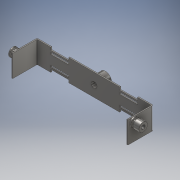
# Autodesk Inventor part: Maintient courvercle
Saved by Autodesk Inventor 2017 (Build 210142000, 142)
## iProperties
Company: FABLAB Frenchmakers
Part Number: Maintient courvercle
Material: Acier inoxydable
Document SubType Name: Modeling
Designer: FABLAB Frenchmakers
Density: 8 g/cm^3
Appearance: Semi-poli
Mass: 121.443 g
Surface Area: 157.681 cm^2
Volume: 15.1804 cm^3
Project: 1400-PopCorn Machine
Stock Number: 1400-01-03
Author: Adrien MARY
Autodesk Inventor part; units mm, degrees
sketch "Esquisse1" plane through (0, 0, 0) normal (0, 0, 1) x (1, 0, 0)
  line L0 (-80, 0) -> (-80, 35)
  line L1 (-80, 35) -> (80, 35)
  line L2 (80, 35) -> (80, 0)
  line L3 (80, 0) -> (78.5, 0)
  line L4 (78.5, 0) -> (78.5, 33.5)
  line L5 (78.5, 33.5) -> (-78.5, 33.5)
  line L6 (-78.5, 33.5) -> (-78.5, 0)
  line L7 (-78.5, 0) -> (-80, 0)
  point P0 (0, 0)
  point P1 (-79.25, 0)
  point P2 (0, 35)
  point P3 (0, 33.5)
  dimension "d0" = 1.5
  dimension "d1" = 1.5
  dimension "d2" = 160
  dimension "d3" = 35
  constraints: 16 end point, 4 vertical, 3 horizontal, 3 midpoint, 2 vertical alignment, 1 collinear, 1 horizontal alignment, 1 perpendicular
  measures "d0" distance between parallel lines of L2 L4
  measures "d1" distance between parallel lines of L1 L5
  measures "d2" distance between parallel lines of L2 L0
  measures "d3" distance between parallel lines of L3 L1
extrude "Extrusion1" add sketch "Esquisse1" along normal mid plane 30
fillet "Congé1" radius 2 2 edges at (80, 35, 0) (-80, 35, 0)
fillet "Congé1" radius 1 2 edges at (-78.5, 33.5, 0) (78.5, 33.5, 0)
sketch "Esquisse2" plane through (-78, 35, 15) normal (0, 1, 0) x (1, 0, 0)
  line L0 (64.3632, 4.6) -> (91.6368, 4.6)
  line L1 (91.6368, 25.4) -> (64.3632, 25.4)
  arc A0 (64.3632, 25.4) -> (64.3632, 4.6) centre (78, 15) ccw
  arc A1 (91.6368, 4.6) -> (91.6368, 25.4) centre (78, 15) ccw
  point P0 (102.0926, 15)
  dimension "d9" = 20.8
  dimension "d10" = 17.15
  dimension "d11" = 17.15
  dimension "d12" = 10.4
  constraints: 4 end point, 4 point on circle, 2 centre point, 1 coincident, 1 horizontal, 1 horizontal alignment, 1 parallel
  measures "d9" distance between parallel lines of L1 L0
  measures "d10" radius of A1
  measures "d11" radius of A0
  measures "d12" distance from line of point (78, 15) L1
extrude "Extrusion2" add sketch "Esquisse2" along normal blind 4
sketch "Esquisse3" plane through (-78, 39, 15) normal (0, 1, 0) x (1, 0, 0)
  circle A0 centre (78, 15) radius 8.75
  dimension "d15" = 17.5
  constraints: 1 centre point, 1 coincident
  measures "d15" diameter of A0
extrude "Extrusion3" add sketch "Esquisse3" along normal blind 10 draft -1.43
sketch "Esquisse6" plane through (-80, 0, -15) normal (-1, 0, 0) x (0, 0, 1)
  circle A0 centre (24, 8) radius 6
  line L0 (30, 33) -> (30, 0) projected
  point P0 (15, 0)
  dimension "d20" = 12
  dimension "d21" = 8
  constraints: 1 centre point, 1 tangent
  measures "d20" diameter of A0
  measures "d21" vertical distance of point (15, 0) A0.centre
extrude "Extrusion4" add sketch "Esquisse6" along normal blind 6.65
ref_plane "Plan de construction4" through (-84.65, 8, 9) normal (-1, 0, 0) x (0, 0, 1)
sketch "Esquisse7" plane through (-84.65, 8, 9) normal (-1, 0, 0) x (0, 0, 1)
  circle A0 centre (0, 0) radius 6 construction
  circle A1 centre (0, 0) radius 3.75
  circle A2 centre (0, 0) radius 7
  point P0 (-9, -8)
  point P1 (6, 0)
  dimension "d25" = 7.5
  dimension "d26" = 1
  constraints: 2 centre point, 2 coincident, 1 horizontal alignment
  measures "d25" diameter of A1
extrude "Extrusion5" cut sketch "Esquisse7" against normal blind 2.6
mirror "Symétrie2" about plane through (0, 0, 0) normal (1, 0, 0) of "Extrusion4", "Extrusion5"
sketch "Esquisse8" plane through (-78, 35, 15) normal (0, 1, 0) x (1, 0, 0)
  line L0 (18.2, 21.5) -> (43, 21.5)
  line L1 (43, 21.5) -> (43, 30)
  line L2 (43, 30) -> (18.2, 30)
  line L3 (18.2, 30) -> (18.2, 21.5)
  line L4 (113, 21.5) -> (137.8, 21.5)
  line L5 (137.8, 21.5) -> (137.8, 30)
  line L6 (137.8, 30) -> (113, 30)
  line L7 (113, 30) -> (113, 21.5)
  line L8 (113, 0) -> (137.8, 0)
  line L9 (137.8, 0) -> (137.8, 8.5)
  line L10 (137.8, 8.5) -> (113, 8.5)
  line L11 (113, 8.5) -> (113, 0)
  line L12 (18.2, 0) -> (43, 0)
  line L13 (43, 0) -> (43, 8.5)
  line L14 (43, 8.5) -> (18.2, 8.5)
  line L15 (18.2, 8.5) -> (18.2, 0)
  line L16 (0, 30) -> (156, 30) projected
  line L17 (156, 0) -> (0, 0) projected
  point P0 (78, 15)
  dimension "d32" = 24.8
  dimension "d33" = 24.8
  dimension "d34" = 70
  dimension "d35" = 35
  dimension "d36" = 8.5
  dimension "d37" = 8.5
  constraints: 32 end point, 8 collinear, 8 parallel, 4 horizontal, 4 perpendicular, 2 point on line
  measures "d32" distance of L13.end L14.end
  measures "d33" distance of L9.end L10.end
  measures "d34" distance between parallel lines of L7 L1
  measures "d35" distance from line of L1 point (78, 15)
  measures "d36" distance between parallel lines of L16 L0
  measures "d37" distance between parallel lines of L17 L14
extrude "Extrusion6" cut sketch "Esquisse8" against normal through all
sketch "Esquisse9" plane through (78, 35, 15) normal (0, 1, 0) x (1, 0, 0)
  line L0 (-137.8, 23.9) -> (-113, 23.9)
  line L1 (-113, 23.9) -> (-113, 26.4)
  line L2 (-113, 26.4) -> (-137.8, 26.4)
  line L3 (-137.8, 26.4) -> (-137.8, 23.9)
  line L4 (-137.8, 3.6) -> (-113, 3.6)
  line L5 (-113, 3.6) -> (-113, 6.1)
  line L6 (-113, 6.1) -> (-137.8, 6.1)
  line L7 (-137.8, 6.1) -> (-137.8, 3.6)
  line L8 (-43, 23.9) -> (-18.2, 23.9)
  line L9 (-18.2, 23.9) -> (-18.2, 26.4)
  line L10 (-18.2, 26.4) -> (-43, 26.4)
  line L11 (-43, 26.4) -> (-43, 23.9)
  line L12 (-43, 3.6) -> (-18.2, 3.6)
  line L13 (-18.2, 3.6) -> (-18.2, 6.1)
  line L14 (-18.2, 6.1) -> (-43, 6.1)
  line L15 (-43, 6.1) -> (-43, 3.6)
  line L16 (-137.8, 21.5) -> (-137.8, 30) projected
  line L17 (-113, 30) -> (-113, 21.5) projected
  line L18 (-43, 21.5) -> (-43, 30) projected
  line L19 (-18.2, 30) -> (-18.2, 21.5) projected
  line L20 (-113, 21.5) -> (-137.8, 21.5) projected
  line L21 (-137.8, 8.5) -> (-113, 8.5) projected
  point P0 (-78, 15)
  dimension "d40" = 2.5
  dimension "d41" = 2.5
  dimension "d42" = 2.4
  dimension "d43" = 2.4
  constraints: 32 end point, 11 collinear, 8 parallel, 4 horizontal, 4 perpendicular, 1 point on line
  measures "d40" distance between parallel lines of L2 L0
  measures "d41" distance between parallel lines of L6 L4
  measures "d42" distance between parallel lines of L20 L0
  measures "d43" distance between parallel lines of L21 L6
extrude "Extrusion7" add sketch "Esquisse9" against normal up to surface (1.5 mm away) contours L3 L2 L1 L0 | L7 L6 L5 L4 | L11 L10 L9 L8 | L15 L14 L13 L12
sketch "Esquisse10" plane through (0, 49, 0) normal (0, 1, 0) x (1, 0, 0)
  point P0 (0, 0)
  point P1 (0, 0)
  constraints: 1 coincident
hole "Perçage1" at (0, 49, 0) direction (0, -1, 0) diameter 8 end through all
ref_plane "Plan de construction5" through (-78, 34.25, 15) normal (0, 1, 0) x (1, 0, 0)
sketch "Esquisse11" plane through (-78, 34.25, 15) normal (0, 1, 0) x (1, 0, 0)
  line L0 (18.2, 23.9) -> (43, 23.9) construction
  line L1 (43, 26.4) -> (18.2, 26.4) construction
  line L2 (18.2, 3.6) -> (43, 3.6) construction
  line L3 (43, 6.1) -> (18.2, 6.1) construction
  line L4 (-59.7354, 25.15) -> (184.2548, 25.15)
  line L5 (-24.0556, 4.85) -> (192.1599, 4.85)
  point P0 (78, 15)
  dimension "d53" = 2.5
  dimension "d54" = 2.5
  dimension "d55" = 1.25
  dimension "d56" = 1.25
  constraints: 4 end point, 2 horizontal
  measures "d53" distance between parallel lines of L1 L0
  measures "d54" distance between parallel lines of L2 L3
  measures "d55" distance between parallel lines of L1 L4
  measures "d56" distance between parallel lines of L2 L5
ref_plane "Plan de construction6" through (86.65, 8, 9) normal (1, 0, 0) x (0, 0, -1)
sketch "Esquisse13" plane through (86.65, 8, 9) normal (1, 0, 0) x (0, 0, -1)
  circle A0 centre (0, 0) radius 6
  circle A1 centre (0, 0) radius 6 construction
  point P0 (9, -8)
  constraints: 1 centre point, 1 coincident, 1 concentric
extrude "Extrusion8" add sketch "Esquisse13" along normal blind 6.5
sketch "Esquisse14" plane through (93.15, 8, 9) normal (1, 0, 0) x (0, 0, -1)
  circle A0 centre (0, 0) radius 6 construction
  point P0 (9, -8)
  constraints: 1 coincident
hole "Perçage2" at (93.15, 8, 9) direction (-1, 0, 0) diameter 4.917 depth 10 tip angle 118 thread size "M6x1" class "6H" standard "ISO Metric profile"
chamfer "Chanfrein2" distance 0.3 angle 45 7 edges at (93.15, 8, 15) (93.15, 8, 11.4585) (84.65, 8, 3) (82.05, 8, 3) (-84.65, 8, 3) (-86.65, 8, 3) (-82.05, 8, 3)
equation "\"d1\" = d0"
equation "\"d11\" = d10"
equation "\"d12\" = 0.5 * d9"
equation "\"d33\" = d32"
equation "\"d35\" = 0.5 * d34"
equation "\"d37\" = d36"
equation "\"d41\" = d40"
equation "\"d43\" = d42"
equation "\"d55\" = 0.5 * d53"
equation "\"d56\" = 0.5 * d54"
equation "\"nombredor\" = 1.61803"
equation "\"pi\" = 3.141593"
